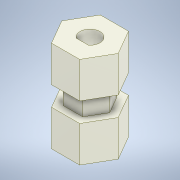
# Autodesk Inventor part: Couple
Saved by Autodesk Inventor 2022 (Build 260153000, 153)
## iProperties
Created: 2021-12-07
Part Number: Couple
Material: Genérico
Document SubType Name: Modeling
Designer: JK
Density: 1 g/cm^3
Appearance: Suave - Marfil
Author: JK
Autodesk Inventor part; units mm, degrees
ref_plane "YZ Plane" through (0, 0, 0) normal (1, 0, 0) x (0, 1, 0)
ref_plane "XZ Plane" through (0, 0, 0) normal (0, 1, 0) x (-1, 0, 0)
ref_plane "XY Plane" through (0, 0, 0) normal (0, 0, 1) x (1, 0, 0)
sketch "Boceto1" plane through (0, 0, 0) normal (0, 1, 0) x (-1, 0, 0)
  line L0 (4.6188, 0) -> (2.3094, -4)
  line L1 (2.3094, -4) -> (-2.3094, -4)
  line L2 (-2.3094, -4) -> (-4.6188, 0)
  line L3 (-4.6188, 0) -> (-2.3094, 4)
  line L4 (-2.3094, 4) -> (2.3094, 4)
  line L5 (2.3094, 4) -> (4.6188, 0)
  circle A0 centre (0, 0) radius 4
  dimension "d0" = 8
  constraints: 12 end point, 1 centre point, 1 coincident, 13 other
  measures "d0" diameter of A0
extrude "Extrusión1" add sketch "Boceto1" along normal blind 15
sketch "Boceto2" plane through (0, 15, 0) normal (0, 1, 0) x (1, 0, 0)
  circle A0 centre (0, 0) radius 1.625
  line L0 (-1.0138, -1.27) -> (1.0138, -1.27)
  dimension "d3" = 3.25
  dimension "d6" = 1.27
  constraints: 2 end point, 2 point on circle, 1 centre point, 1 coincident, 1 horizontal
  measures "d3" diameter of A0
  measures "d6" distance from line of point (0, 0) L0
extrude "Extrusión2" cut sketch "Boceto2" against normal blind 7 contours A0 L0 picked at (0.4054, -0.3153)
sketch "Boceto3" plane through (0, 0, 0) normal (0, -1, 0) x (1, 0, 0)
  circle A0 centre (0, 0) radius 0.825
  dimension "d7" = 1.65
  constraints: 1 centre point, 1 coincident
  measures "d7" diameter of A0
extrude "Extrusión3" cut sketch "Boceto3" against normal blind 7
sketch "Boceto4" plane through (0, 7, 0) normal (0, -1, 0) x (1, 0, 0)
  circle A0 centre (0, 0) radius 0.825 projected
  line L0 (0, -0.825) -> (0, 0.825)
  circle A1 centre (0, 0) radius 0.825 projected
  constraints: 2 end point, 2 point on circle, 1 midpoint, 1 vertical
extrude "Extrusión4" add sketch "Boceto4" along normal blind 1.5 contours A0 L0 picked at (0.215, 0.1715)
ref_plane "Plano de trabajo1" through (0, 7.5, 0) normal (0, 1, 0) x (1, 0, 0)
sketch "Boceto5" plane through (0, 7.5, 0) normal (0, 1, 0) x (1, 0, 0)
  circle A0 centre (0, 0) radius 0.825 projected
  line L0 (4.6188, 0) -> (2.3094, 4) projected
  line L1 (2.3094, -4) -> (4.6188, 0) projected
  line L2 (-2.3094, -4) -> (2.3094, -4) projected
  line L3 (-4.6188, 0) -> (-2.3094, -4) projected
  line L4 (-2.3094, 4) -> (-4.6188, 0) projected
  line L5 (2.3094, 4) -> (-2.3094, 4) projected
  line L6 (-3.2332, 0) -> (-1.6166, -2.8)
  line L7 (-1.6166, -2.8) -> (1.6166, -2.8)
  line L8 (1.6166, -2.8) -> (3.2332, 0)
  line L9 (3.2332, 0) -> (1.6166, 2.8)
  line L10 (1.6166, 2.8) -> (-1.6166, 2.8)
  line L11 (-1.6166, 2.8) -> (-3.2332, 0)
  arc A1 (0, 0.825) -> (0, -0.825) centre (0, 0) ccw projected
  circle A2 centre (0, 0) radius 6.7948
  dimension "d13" = 1.2
  constraints: 12 end point, 1 centre point, 1 coincident, 5 other
  measures "d13" distance between parallel lines of L4 L11
extrude "Extrusión5" cut sketch "Boceto5" along normal mid plane 3.2 contours L1 L2 L3 L4 L5 L0
